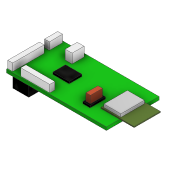
# Autodesk Inventor part: Nordic_PCB
Saved by Autodesk Inventor 2022.3 (Build 263350000, 350)
## iProperties
Created: 2023-07-18
Part Number: Nordic_PCB
Material: Genérico
Document SubType Name: Modeling
Designer: Usuario
Density: 1 g/cm^3
Appearance: Valor por defecto
Author: Usuario
Autodesk Inventor part; units mm, degrees
ref_plane "YZ Plane" through (0, 0, 0) normal (1, 0, 0) x (0, 1, 0)
ref_plane "XZ Plane" through (0, 0, 0) normal (0, 1, 0) x (-1, 0, 0)
ref_plane "XY Plane" through (0, 0, 0) normal (0, 0, 1) x (1, 0, 0)
sketch "Boceto1" plane through (0, 0, 0) normal (0, 1, 0) x (-1, 0, 0)
  line L0 (-25, 13.15) -> (25, 13.15)
  line L1 (25, 13.15) -> (25, -13.15)
  line L2 (25, -13.15) -> (-25, -13.15)
  line L3 (-25, -13.15) -> (-25, 13.15)
  line L4 (-25, 13.15) -> (25, -13.15) construction
  line L5 (25, 13.15) -> (-25, -13.15) construction
  point P0 (0, 0)
  dimension "d0" = 50
  dimension "d1" = 26.3
  constraints: 12 end point, 2 midpoint, 2 parallel, 1 horizontal, 1 perpendicular
  measures "d0" distance of L1.end L2.end
  measures "d1" distance of L0.end L1.end
extrude "Extrusión1" add sketch "Boceto1" along normal blind 1.6
sketch "Boceto2" plane through (0, 1.6, 0) normal (0, 1, 0) x (1, 0, 0)
  line L0 (15.6711, -6.5623) -> (32.2824, -6.5623)
  line L1 (32.2824, -6.5623) -> (32.2824, 6.5623)
  line L2 (32.2824, 6.5623) -> (15.6711, 6.5623)
  line L3 (15.6711, 6.5623) -> (15.6711, -6.5623)
  line L4 (15.6711, -6.5623) -> (32.2824, 6.5623) construction
  line L5 (32.2824, -6.5623) -> (15.6711, 6.5623) construction
  point P0 (0, 0)
  point P1 (23.9767, 0)
  constraints: 12 end point, 2 midpoint, 2 parallel, 1 horizontal, 1 perpendicular
extrude "Extrusión2" add sketch "Boceto2" along normal blind 0.5
sketch "Boceto3" plane through (0, 2.1, 0) normal (0, 1, 0) x (1, 0, 0)
  line L0 (24.9953, -5.8962) -> (16.4546, -5.8962)
  line L1 (16.4546, -5.8962) -> (16.4546, 5.8962)
  line L2 (16.4546, 5.8962) -> (24.9953, 5.8962)
  line L3 (24.9953, 5.8962) -> (24.9953, -5.8962)
  line L4 (24.9953, -5.8962) -> (16.4546, 5.8962) construction
  line L5 (16.4546, -5.8962) -> (24.9953, 5.8962) construction
  point P0 (0, 0)
  point P1 (20.725, 0)
  constraints: 12 end point, 2 midpoint, 2 parallel, 1 horizontal, 1 perpendicular
extrude "Extrusión3" add sketch "Boceto3" along normal blind 1.5
sketch "Boceto4" plane through (0, 1.6, 0) normal (0, 1, 0) x (1, 0, 0)
  line L0 (-24.7819, -12.6535) -> (-22.3667, -12.6535)
  line L1 (-22.3667, -12.6535) -> (-22.3667, 3.0977)
  line L2 (-22.3667, 3.0977) -> (-24.7819, 3.0977)
  line L3 (-24.7819, 3.0977) -> (-24.7819, -12.6535)
  line L4 (-24.7819, 5.6879) -> (-22.3667, 5.6879)
  line L5 (-22.3667, 5.6879) -> (-22.3667, 12.3034)
  line L6 (-22.3667, 12.3034) -> (-24.7819, 12.3034)
  line L7 (-24.7819, 12.3034) -> (-24.7819, 5.6879)
  line L8 (-18.3064, -12.6535) -> (-7.2456, -12.6535)
  line L9 (-7.2456, -12.6535) -> (-7.2456, -10.0983)
  line L10 (-7.2456, -10.0983) -> (-18.3064, -10.0983)
  line L11 (-18.3064, -10.0983) -> (-18.3064, -12.6535)
  line L12 (-7.2456, -12.6535) -> (-3.8465, -12.6535)
  line L13 (-3.8465, -12.6535) -> (-3.8465, -10.0983)
  line L14 (-3.8465, -10.0983) -> (-7.2456, -10.0983)
  line L15 (-7.2456, -10.0983) -> (-7.2456, -12.6535)
  point P0 (0, 0)
  constraints: 32 end point, 8 parallel, 4 horizontal, 4 perpendicular, 4 point on line
extrude "Extrusión4" add sketch "Boceto4" along normal blind 3.7
sketch "Boceto5" plane through (0, 1.6, 0) normal (0, 1, 0) x (1, 0, 0)
  line L0 (9.1061, -9.0184) -> (12.7089, -9.0184)
  line L1 (12.7089, -9.0184) -> (12.7089, -1.3991)
  line L2 (12.7089, -1.3991) -> (9.1061, -1.3991)
  line L3 (9.1061, -1.3991) -> (9.1061, -9.0184)
  line L4 (-11.1445, -3.83) -> (-2.9401, -3.83)
  line L5 (-2.9401, -3.83) -> (-2.9401, 2.5512)
  line L6 (-2.9401, 2.5512) -> (-11.1445, 2.5512)
  line L7 (-11.1445, 2.5512) -> (-11.1445, -3.83)
  point P0 (0, 0)
  constraints: 16 end point, 4 parallel, 2 horizontal, 2 perpendicular
extrude "Extrusión5" add sketch "Boceto5" along normal blind 1
sketch "Boceto6" plane through (0, 1.6, 0) normal (0, 1, 0) x (1, 0, 0)
  line L0 (-14.2306, 5.4877) -> (-10.7922, 5.4877)
  line L1 (-10.7922, 5.4877) -> (-10.7922, 11.4752)
  line L2 (-10.7922, 11.4752) -> (-14.2306, 11.4752)
  line L3 (-14.2306, 11.4752) -> (-14.2306, 5.4877)
  point P0 (0, 0)
  constraints: 8 end point, 2 parallel, 1 horizontal, 1 perpendicular
extrude "Extrusión6" add sketch "Boceto6" along normal blind 4.7
sketch "Boceto7" plane through (0, 2.6, 0) normal (0, 1, 0) x (1, 0, 0)
  line L0 (9.8007, -8.1731) -> (12.0409, -8.1731)
  line L1 (12.0409, -8.1731) -> (12.0409, -2.1527)
  line L2 (12.0409, -2.1527) -> (9.8007, -2.1527)
  line L3 (9.8007, -2.1527) -> (9.8007, -8.1731)
  point P0 (0, 0)
  constraints: 8 end point, 2 parallel, 1 horizontal, 1 perpendicular
extrude "Extrusión7" add sketch "Boceto7" along normal blind 3.7
sketch "Boceto8" plane through (0, 0, 0) normal (0, -1, 0) x (1, 0, 0)
  line L0 (-25, -13.15) -> (-25, 13.15) projected
  line L1 (-25, 0) -> (-22.5, 0)
  line L2 (-22.5, 0) -> (-22.5, -12.5)
  line L3 (-22.5, -12.5) -> (-14.5, -12.5)
  line L4 (-24.7819, -12.3034) -> (-22.3667, -12.3034) projected
  line L5 (-22.5, -12.5) -> (-14.5, -12.5) construction
  line L6 (-14.5, -12.5) -> (-14.5, 12.5)
  line L7 (-14.5, 12.5) -> (-22.5, 12.5)
  line L8 (-25, 13.15) -> (25, 13.15) projected
  line L9 (-22.5, 12.5) -> (-22.5, 0)
  point P0 (0, 0)
  dimension "d16" = 2.5
  dimension "d17" = 12.5
  dimension "d18" = 8
  dimension "d19" = 0
  dimension "d20" = 25
  constraints: 14 end point, 3 perpendicular, 2 horizontal, 2 parallel, 1 collinear, 1 midpoint
  measures "d16" distance of L1.start L1.end
  measures "d17" distance of L1.end L2.end
  measures "d18" distance of L2.end L3.end
  measures "d19" distance between parallel lines of L3 L5
  measures "d20" distance of L3.end L6.end
extrude "Extrusión8" add sketch "Boceto8" along normal blind 5.7
